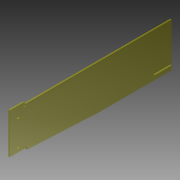
# Autodesk Inventor part: window
Saved by Autodesk Inventor 2014 SP2 (Build 180246200, 246)
## iProperties
Created: 2016-05-05
Part Number: window
Material: Generic
Document SubType Name: Modeling
Designer: cruiser
Density: 1 g/cm^3
Appearance: Clear - Yellow
Author: cruiser
Autodesk Inventor part; units mm, degrees
ref_plane "YZ Plane" through (0, 0, 0) normal (1, 0, 0) x (0, 1, 0)
ref_plane "XZ Plane" through (0, 0, 0) normal (0, 1, 0) x (-1, 0, 0)
ref_plane "XY Plane" through (0, 0, 0) normal (0, 0, 1) x (1, 0, 0)
sketch "Sketch2" plane through (0, 0, 0) normal (1, 0, 0) x (0, 1, 0)
  line L0 (167.4563, -46.0313) -> (-167.4563, -46.0312)
  line L1 (-167.4563, -46.0312) -> (-167.4563, 46.0313)
  line L2 (-167.4563, 46.0313) -> (167.4563, 46.0312)
  line L3 (167.4563, 46.0312) -> (167.4563, -46.0313)
  line L4 (167.4563, -46.0313) -> (-167.4563, 46.0313) construction
  line L5 (-167.4563, -46.0312) -> (167.4563, 46.0312) construction
  line L6 (-167.4563, 41.0312) -> (-214.9238, 41.0312)
  line L7 (-214.9238, 41.0312) -> (-214.9238, -42.8563)
  line L8 (-214.9238, -42.8563) -> (-167.4562, -42.8563)
  line L9 (-167.4562, -42.8563) -> (-167.4563, 41.0312)
  line L10 (167.4563, -46.0313) -> (0, -46.0312)
  line L11 (0, -46.0312) -> (0, -56.0312)
  line L12 (0, -56.0312) -> (167.4563, -56.0312)
  line L13 (167.4563, -56.0312) -> (167.4563, -46.0313)
  line L14 (0, 0) -> (0, -46.0312)
  line L15 (-167.4563, 46.0313) -> (-170.6312, 46.0313)
  line L16 (-170.6312, 46.0313) -> (-170.6312, 41.0312)
  line L17 (-170.6312, 41.0312) -> (-167.4563, 41.0312)
  line L18 (-167.4563, 41.0312) -> (-167.4563, 46.0313)
  line L19 (-214.9238, 41.0312) -> (-172.695, 41.0312)
  line L20 (-172.695, 41.0312) -> (-172.695, 46.0312)
  line L21 (-172.695, 46.0312) -> (-214.9238, 46.0312)
  line L22 (-214.9238, 46.0312) -> (-214.9238, 41.0312)
  line L23 (-214.9238, 46.0312) -> (-174.695, 46.0312)
  line L24 (-174.695, 46.0312) -> (-174.695, 51.0312)
  line L25 (-174.695, 51.0312) -> (-214.9238, 51.0312)
  line L26 (-214.9238, 51.0312) -> (-214.9238, 46.0312)
  line L27 (-172.695, 46.0312) -> (-174.695, 51.0312)
  line L28 (-167.4563, -46.0312) -> (0, -46.0312)
  line L29 (0, -46.0312) -> (0, -47.6188)
  line L30 (0, -47.6188) -> (-167.4563, -47.6188)
  line L31 (-167.4563, -47.6188) -> (-167.4563, -46.0312)
  line L32 (0, -56.0312) -> (-167.4563, -47.6188)
  dimension "d0" = 334.9125
  dimension "d1" = 92.0625
  dimension "d6" = 3.175
  dimension "d7" = 5
  dimension "d8" = 47.4675
  dimension "d9" = 10
  dimension "d17" = 0
  dimension "d18" = 3.175
  dimension "d19" = 2.0638
  dimension "d20" = 5
  dimension "d21" = 2
  dimension "d22" = 1.5875
  constraints: 66 end point, 14 parallel, 7 horizontal, 7 perpendicular, 3 midpoint, 2 collinear, 2 point on line
  measures "d0" distance of L1.end L2.end
  measures "d1" distance of L0.end L1.end
  measures "d6" distance between parallel lines of L0 L8
  measures "d7" distance between parallel lines of L2 L6
  measures "d8" distance between parallel lines of L1 L7
  measures "d9" distance between parallel lines of L0 L12
  measures "d17" distance between parallel lines of L14 L11
  measures "d18" distance of L1.end L15.end
  measures "d19" distance between parallel lines of L16 L20
  measures "d20" distance of L25.end L21.end
  measures "d21" distance between parallel lines of L20 L24
  measures "d22" distance between parallel lines of L28 L30
extrude "Extrusion1" add sketch "Sketch2" along normal blind 3.15
sketch "Sketch3" plane through (3.15, 0, 0) normal (1, 0, 0) x (0, 0, -1)
  line L0 (56.0312, 0) -> (56.0312, 167.4563) projected
  line L1 (56.0312, 167.4563) -> (-46.0312, 167.4563) projected
  line L2 (42.8812, 167.4563) -> (46.0312, 167.4563)
  line L3 (46.0312, 167.4563) -> (46.0312, 127.4563)
  line L4 (46.0312, 127.4563) -> (42.8813, 127.4563)
  line L5 (42.8813, 127.4563) -> (42.8812, 167.4563)
  line L6 (-41.0312, -170.6312) -> (-41.0312, -172.695) projected
  line L7 (-51.0312, -214.9238) -> (42.8563, -214.9238) projected
  circle A0 centre (-26.2562, -191.19) radius 2.5
  line L8 (47.6188, -167.4563) -> (-41.0312, -167.4563)
  line L9 (-41.0312, -167.4563) -> (-41.0312, -214.9238)
  line L10 (-41.0312, -214.9238) -> (47.6188, -214.9237)
  line L11 (47.6188, -214.9237) -> (47.6188, -167.4563)
  line L12 (3.2938, -214.9238) -> (3.2938, -167.4563)
  circle A1 centre (32.8438, -191.19) radius 2.5
  point P0 (0, 0)
  dimension "d11" = 40
  dimension "d12" = 3.15
  dimension "d13" = 10
  dimension "d23" = 5
  dimension "d24" = 23.7338
  dimension "d25" = 29.55
  constraints: 18 end point, 4 parallel, 2 centre point, 2 horizontal, 2 midpoint, 2 perpendicular, 2 point on line, 1 collinear, 1 symmetric about line, 1 other
  measures "d11" distance of L4.end L2.start
  measures "d12" distance between parallel lines of L3 L5
  measures "d13" distance between parallel lines of L0 L3
  measures "d23" diameter of A0
  measures "d24" distance from line of A0.centre L7
  measures "d25" distance from line of L12 A0.centre
extrude "Extrusion2" cut sketch "Sketch3" against normal blind 10 contours L3 L4 L5 L1 | A0 | A1
equation "\"d0\" = window_z"
equation "\"d1\" = window_y"
equation "\"d6\" = 2 * sm_thickness"
equation "\"d7\" = acrylic_into_frame"
equation "\"d8\" = window_overlap"
equation "\"d9\" = protection_slot_width"
equation "\"d18\" = 2 * sm_thickness"
equation "\"d19\" = 1.3 * sm_thickness"
equation "\"d22\" = sm_thickness"
equation "\"d2\" = clear_acrylic"
equation "\"d11\" = 0.5 * protection_slot_length"
equation "\"d12\" = clear_acrylic"
equation "\"d13\" = protection_slot_width"
equation "\"d23\" = m5_diameter"
equation "\"d24\" = 0.5 * window_overlap"
equation "\"d25\" = 0.333333 * drawer_y"
equation "\"sm_thickness\" = 1.5875"
equation "\"very_thick_acrylic\" = 9.45"
equation "\"thick_acrylic\" = 5.88"
equation "\"thin_acrylic\" = 3.15"
equation "\"clear_acrylic\" = 3.15"
equation "\"wood_thickness\" = 6.72"
equation "\"m3_diameter\" = 3"
equation "\"m4_diameter\" = 4"
equation "\"m5_diameter\" = 5"
equation "\"brass_insert_drill\" = 4"
equation "\"m5_brass_insert_drill\" = 6.7"
equation "\"m3_main_length\" = 14"
equation "\"m3_main_nut_width\" = 5.7"
equation "\"m3_main_nut_thickness\" = 2.5"
equation "\"m3_main_extra\" = 1"
equation "\"stepper_screw_space\" = 35"
equation "\"stepper_shaft_diameter\" = 5"
equation "\"stepper_body_diameter\" = 28"
equation "\"laser_body_diameter\" = 12"
equation "\"carrier_y\" = 251"
equation "\"carrier_z\" = 12"
equation "\"visor_x\" = 257.3"
equation "\"visor_y\" = 110.2375"
equation "\"protection_slot\" = 44.2"
equation "\"protection_slot_offset\" = 55.25"
equation "\"window_z\" = 334.9125"
equation "\"tray_border\" = 25"
equation "\"bed_z2\" = 79.6"
equation "\"bed_z\" = 25.4"
equation "\"reservoir_x\" = 201"
equation "\"crane_z2\" = 12"
equation "\"tray_y\" = 251"
equation "\"door_sensor\" = 35"
equation "\"linear_bearing_spacing\" = 267"
equation "\"motor_spacing\" = 337"
equation "\"tray_x\" = 251"
equation "\"reservoir_y\" = 201"
equation "\"window_y\" = 92.0625"
equation "\"end_stop_spacing\" = 19"
equation "\"window_overlap\" = 47.4675"
equation "\"door_z\" = 334.9125"
equation "\"door_x\" = 251"
equation "\"door_overlap\" = 47.4675"
equation "\"acrylic_into_frame\" = 5"
equation "\"protection_slot_width\" = 10"
equation "\"laser_z_offset\" = 55"
equation "\"galvo_frame_x\" = 66"
equation "\"galvo_frame_z\" = 65"
equation "\"laser_y_offset\" = 19.4"
equation "\"thumb_nut_diameter\" = 7"
equation "\"drawer_y\" = 88.65"
equation "\"frame_total_z\" = 661"
equation "\"printer_z\" = 289"
equation "\"subframe_y_offset\" = 27.5"
equation "\"frame_bottom_z\" = 275"
equation "\"lcd_y\" = 25"
equation "\"drawer_x\" = 257.3"
equation "\"drawer_z\" = 278.175"
equation "\"drawer_z_from_bottom\" = 25"
equation "\"t_galvo_frame\" = 6.72"
equation "\"laser_x\" = 24"
equation "\"laser_z\" = 18"
equation "\"nema17_x\" = 43"
equation "\"thumb_nut_offset_y\" = 0"
equation "\"laser_y\" = 35"
equation "\"frame_tilt\" = 1deg"
equation "\"frame_top_z\" = 386"
equation "\"frame_border\" = 46.35"
equation "\"laser_diameter\" = 12"
equation "\"galvo_frame_y_offset\" = 27.5"
equation "\"lcd_x\" = 72"
equation "\"subframe_x\" = 195"
equation "\"frame_foot_z\" = 12"
equation "\"z_min_from_center\" = 115"
equation "\"m3_press_nut_drill\" = 4.5"
equation "\"m3_head\" = 6"
equation "\"m5_press_nut_drill\" = 6.5"
equation "\"drawer_support_from_top\" = 47.4675"
equation "\"protection_slot_length\" = 80"
body "Solid1"
